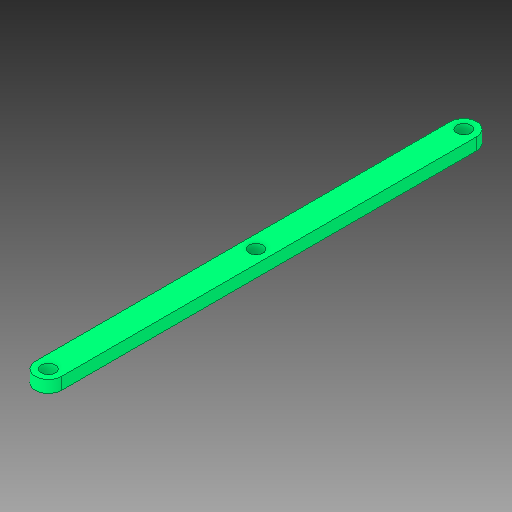
# Autodesk Inventor part: 阿克曼長軸
Saved by Autodesk Inventor 2019 (Build 230136000, 136)
## iProperties
Created: 2020-03-15
Part Number: 阿克曼長軸
Material: 一般
Document SubType Name: Modeling
Designer: 吳昇峻
Density: 1 g/cm^3
Appearance: 預設
Author: 吳昇峻
Autodesk Inventor part; units mm, degrees
ref_plane "YZ Plane" through (0, 0, 0) normal (1, 0, 0) x (0, 1, 0)
ref_plane "XZ Plane" through (0, 0, 0) normal (0, 1, 0) x (-1, 0, 0)
ref_plane "XY Plane" through (0, 0, 0) normal (0, 0, 1) x (1, 0, 0)
sketch "草圖1" plane through (0, 0, 0) normal (0, 1, 0) x (-1, 0, 0)
  arc A0 (3.25, -9) -> (-3.25, -9) centre (0, -9) ccw
  circle A1 centre (0, -9) radius 1.75
  line L0 (0, -9) -> (0, -60.5) construction
  circle A2 centre (0, -60.5) radius 1.75
  line L1 (0, -60.5) -> (0, -112) construction
  circle A3 centre (0, -112) radius 1.75
  arc A4 (-3.25, -112) -> (3.25, -112) centre (0, -112) ccw
  line L2 (3.25, -9) -> (3.25, -112)
  line L3 (-3.25, -9) -> (-3.25, -112)
  dimension "d1" = 6.5
  dimension "d2" = 3.5
  dimension "d8" = 51.5
  dimension "d9" = 3.5
  dimension "d12" = 51.5
  dimension "d13" = 3.5
  dimension "d14" = 6.5
  constraints: 8 end point, 5 centre point, 4 coincident, 4 point on circle, 3 vertical, 1 tangent
  measures "d1" diameter of A0
  measures "d2" diameter of A1
  measures "d8" distance of L0.start L0.end
  measures "d9" diameter of A2
  measures "d12" distance of L1.start L1.end
  measures "d13" diameter of A3
  measures "d14" diameter of A4
extrude "擠出3" add sketch "草圖1" along normal blind 3
